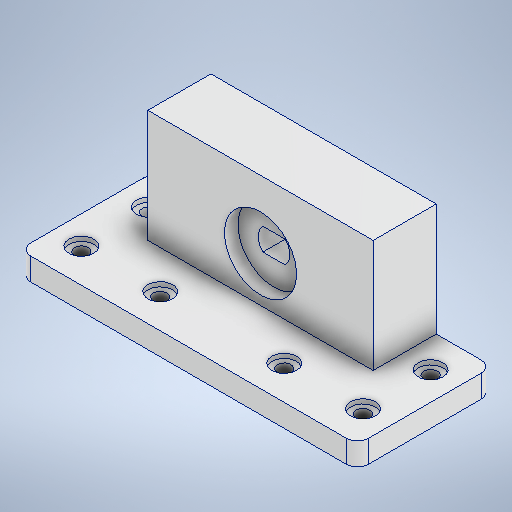
# Autodesk Inventor part: motor_bracket
Saved by Autodesk Inventor 2026.2 (Build 302298010, 298A)
## iProperties
Created: 2026-03-27
Part Number: motor_bracket
Material: Aluminum 6061
Document SubType Name: Modeling
Designer: chanh
Density: 2.7 g/cm^3
Appearance: Aluminum - Flat
Author: chanh
Autodesk Inventor part; units mm, degrees
ref_plane "YZ Plane" through (0, 0, 0) normal (1, 0, 0) x (0, 1, 0)
ref_plane "XZ Plane" through (0, 0, 0) normal (0, 1, 0) x (-1, 0, 0)
ref_plane "XY Plane" through (0, 0, 0) normal (0, 0, 1) x (1, 0, 0)
sketch "Sketch1" plane through (0, 0, 0) normal (0, 0, 1) x (1, 0, 0)
  circle A0 centre (0, 0) radius 7
  line L0 (-4.95, 4.9495) -> (4.95, 4.9495)
  line L1 (-4.95, -4.9495) -> (4.95, -4.9495)
  line L2 (0, 0) -> (0, -30) construction
  line L3 (-75, -30) -> (75, -30)
  line L4 (75, -30) -> (75, -20)
  line L5 (75, -20) -> (-75, -20)
  line L6 (-75, -20) -> (-75, -30)
  line L7 (-75, -30) -> (75, -20) construction
  line L8 (75, -30) -> (-75, -20) construction
  line L9 (-50, -20) -> (50, -20)
  line L10 (50, -20) -> (50, 30)
  line L11 (50, 30) -> (-50, 30)
  line L12 (-50, 30) -> (-50, -20)
  point P0 (0, -25)
  dimension "d1" = 7
  dimension "d2" = 9.9
  dimension "d4" = 150
  dimension "d5" = 10
  dimension "d6" = 50
  dimension "d26" = 25
  dimension "d27" = 100
  dimension "d28" = 50
  constraints: 26 end point, 5 parallel, 4 point on circle, 3 horizontal, 2 coincident, 2 midpoint, 2 perpendicular, 2 point on line, 1 centre point, 1 vertical, 1 vertical alignment
  measures "d1" radius of A0
  measures "d2" distance of L0.start L0.end
  measures "d4" distance of L3.start L3.end
  measures "d5" distance of L5.end L3.start
  measures "d6" distance from line of L9.start L2
  measures "d26" distance of point (0, -25) point (0, 0)
  measures "d27" distance of L11.end L10.end
  measures "d28" distance of L10.end L9.end
extrude "Extrusion1" add sketch "Sketch1" along normal blind 28 contours L0 A0 | A0 L1 | L6 L5 L4 L3 | L12 L11 L10 L5
sketch "Sketch2" plane through (0, 0, 28) normal (0, 0, 1) x (1, 0, 0)
  line L0 (-50, -20) -> (-75, -20) projected
  line L1 (-75, -20) -> (-75, -30) projected
  line L2 (-75, -30) -> (75, -30) projected
  line L3 (75, -30) -> (75, -20) projected
  line L4 (-50, -20) -> (50, -20)
  line L5 (75, -20) -> (50, -20) projected
  line L6 (50, -20) -> (50, 30) projected
  line L7 (50, 30) -> (-50, 30) projected
  line L8 (-50, 30) -> (-50, -20) projected
  point P0 (0, 0)
  constraints: 2 end point
extrude "Extrusion2" add sketch "Sketch2" along normal blind 32 contours L4 L5 L3 L2 L1 L0
sketch "Sketch3" plane through (0, 0, 60) normal (0, 0, 1) x (1, 0, 0)
  circle A0 centre (0, 0) radius 16
  dimension "d11" = 32
  constraints: 1 centre point, 1 coincident
  measures "d11" diameter of A0
extrude "Extrusion3" cut sketch "Sketch3" against normal blind 38
sketch "Sketch4" plane through (-75, -20, 0) normal (0, 1, 0) x (1, 0, 0)
  circle A0 centre (12.5, -15) radius 3.05
  line L0 (150, 0) -> (0, 0) projected
  circle A1 centre (12.5, -45) radius 3.05
  circle A2 centre (47.5, -45) radius 3.05
  line L1 (75, 12) -> (75, -72) projected
  circle A3 centre (137.5, -15) radius 3.05
  circle A4 centre (137.5, -45) radius 3.05
  circle A5 centre (102.5, -45) radius 3.05
  line L2 (0, 0) -> (0, -60) projected
  point P0 (75, 0)
  point P1 (25, 0)
  point P2 (12.5, 0)
  point P3 (12.5, 0)
  point P4 (12.5, 0)
  point P5 (12.5, 0)
  dimension "d14" = 6.1
  dimension "d15" = 15
  dimension "d17" = 30
  dimension "d18" = 35
  constraints: 6 centre point, 3 point on line, 3 symmetric about line, 2 equal radius, 2 vertical alignment, 1 coincident, 1 horizontal alignment, 3 other
  measures "d14" diameter of A0
  measures "d15" distance of A0.centre point (12.5, 0)
  measures "d17" distance of A1.centre A0.centre
  measures "d18" distance of A2.centre A1.centre
extrude "Extrusion4" cut sketch "Sketch4" against normal through all
fillet "Fillet1" radius 5 4 edges at (75, -25, 60) (-75, -25, 60) (75, -25, 0) (-75, -25, 0)
sketch "Sketch5" plane through (-50, -20, 28) normal (0, 1, 0) x (1, 0, 0)
  arc A0 (-20, 28) -> (-25, 23) centre (-20, 23) ccw projected
  line L0 (-25, 23) -> (-25, -27) projected
  line L1 (0, 28) -> (-20, 28) projected
  circle A1 centre (-12.5, 13) radius 3.05 projected
  circle A2 centre (112.5, 13) radius 3.05 projected
  arc A3 (125, 23) -> (120, 28) centre (120, 23) ccw projected
  line L2 (125, 23) -> (125, -27) projected
  circle A4 centre (-12.5, 13) radius 5.5
  circle A5 centre (-12.5, -17) radius 5.5
  circle A6 centre (22.5, -17) radius 5.5
  circle A7 centre (77.5, -17) radius 5.5
  circle A8 centre (112.5, -17) radius 5.5
  circle A9 centre (112.5, 13) radius 5.5
  arc A10 (-20, 28) -> (-25, 23) centre (-20, 23) ccw projected
  line L3 (-25, 23) -> (-25, -27) projected
  arc A11 (-25, -27) -> (-20, -32) centre (-20, -27) ccw projected
  line L4 (120, -32) -> (-20, -32) projected
  arc A12 (120, -32) -> (125, -27) centre (120, -27) ccw projected
  arc A13 (-25, -27) -> (-20, -32) centre (-20, -27) ccw projected
  line L5 (120, -32) -> (-20, -32) projected
  arc A14 (120, -32) -> (125, -27) centre (120, -27) ccw projected
  line L6 (125, 23) -> (125, -27) projected
  arc A15 (125, 23) -> (120, 28) centre (120, 23) ccw projected
  circle A16 centre (-12.5, -17) radius 3.05 projected
  circle A17 centre (22.5, -17) radius 3.05 projected
  circle A18 centre (77.5, -17) radius 3.05 projected
  circle A19 centre (112.5, -17) radius 3.05 projected
  line L7 (0, 28) -> (0, 0) projected
  line L8 (0, 28) -> (-20, 28) projected
  line L9 (120, 28) -> (100, 28) projected
  line L10 (100, 28) -> (100, 0) projected
  line L11 (0, 28) -> (0, 0) projected
  line L12 (120, 28) -> (100, 28) projected
  line L13 (100, 28) -> (100, 0) projected
  line L14 (0, 0) -> (100, 0) projected
  line L15 (0, 0) -> (100, 0) projected
  point P0 (50, 28)
  dimension "d22" = 11
  constraints: 6 centre point, 6 coincident, 5 equal radius
  measures "d22" diameter of A4
extrude "Extrusion5" cut sketch "Sketch5" against normal blind 2 contours A1 | A2 | A4 | A5 | A6 | A7 | A8 | A9 | A16 | A17 | A18 | A19
body "Solid1"
